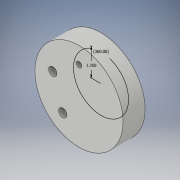
# Autodesk Inventor part: ArthurW5.5aHoles
Saved by Autodesk Inventor 2018 (Build 220112000, 112)
## iProperties
Created: 2019-01-14
Part Number: ArthurW5.5aHoles
Material: Generic
Document SubType Name: Modeling
Designer: This kid
Density: 1 g/cm^3
Appearance: Default
Author: This kid
Autodesk Inventor part; units mm, degrees
ref_plane "YZ Plane" through (0, 0, 0) normal (1, 0, 0) x (0, 1, 0)
ref_plane "XZ Plane" through (0, 0, 0) normal (0, 1, 0) x (-1, 0, 0)
ref_plane "XY Plane" through (0, 0, 0) normal (0, 0, 1) x (1, 0, 0)
sketch "Sketch1" plane through (0, 0, 0) normal (0, 0, 1) x (1, 0, 0)
  circle A0 centre (0, 0) radius 50.8
  circle A1 centre (0, 0) radius 31.75
  dimension "d0" = 101.6
  dimension "d1" = 63.5
  constraints: 2 centre point, 2 coincident
  measures "d0" diameter of A0
  measures "d1" diameter of A1
extrude "Extrusion2" add sketch "Sketch1" along normal blind 25.4 contours A0 | A1
sketch "Sketch4" plane through (0, 0, 0) normal (0, 0, -1) x (-1, 0, 0)
  point P0 (0, 0)
  point P1 (0, 31.75)
  point P2 (-30.196, 9.8113)
  point P3 (0, 0)
  point P4 (-18.6622, -25.6863)
  point P5 (0, 0)
  point P6 (18.6622, -25.6863)
  point P7 (0, 0)
  point P8 (30.196, 9.8113)
  point P9 (0, 0)
  dimension "d12" = 31.75
  dimension "d15" = 360
  constraints: 2 coincident, 9 other
  measures "d12" distance of point (0, 0) point (0, 31.75)
hole "Hole1" at (0, 31.75, 0) direction (0, 0, 1) diameter 6.35 end through all
hole "Hole2" at (-30.196, 9.8113, 0) at (-18.6622, -25.6863, 0) direction (0, 0, 1) diameter 9.525 end through all counterbore diameter 19.05 counterbore depth 6.35
hole "Hole3" at (18.6622, -25.6863, 0) direction (0, 0, 1) diameter 4.9784 depth 19.05 thread size "1/4-20 UNC" class "1B" standard "ANSI Unified Screw Threads"
hole "Hole4" at (30.196, 9.8113, 0) direction (0, 0, 1) diameter 13.4874 depth 19.05 clearance for "Hex Head Bolt" size "1/2" standard "Ansi Unified Screw Threads"
equation "\"d22\" = d12"
equation "\"d29\" = d12"
body "Solid2"
